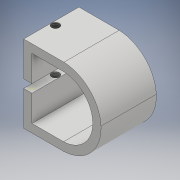
# Autodesk Inventor part: Goupille
Saved by Autodesk Inventor 2018.1 (Build 221171000, 171)
## iProperties
Created: 2019-11-08
Part Number: Goupille
Material: Générique
Document SubType Name: Modeling
Designer: tgremling1
Density: 1 g/cm^3
Appearance: Par défaut
Author: tgremling1
Autodesk Inventor part; units mm, degrees
ref_plane "YZ Plane" through (0, 0, 0) normal (1, 0, 0) x (0, 1, 0)
sketch "Esquisse1" plane through (0, 0, 0) normal (0, 1, 0) x (-1, 0, 0)
  line L0 (11, -11) -> (11, 11)
  arc A0 (-0.5, 11) -> (-11, -0.5) centre (-0.0119, 0.0108) ccw
  arc A1 (-11, 0.5) -> (0, -11) centre (-0.0114, 0) ccw
  line L1 (11, 11) -> (-0.5, 11)
  line L2 (11, -11) -> (-0.5, -11)
  arc A2 (-0.5626, 14) -> (-13.9968, -0.6393) centre (-0.0119, 0.0108) ccw
  line L3 (-0.5626, 14) -> (14, 14)
  line L4 (14, 14) -> (14, -14)
  line L5 (14, -14) -> (-0.5, -14)
  arc A3 (-13.9968, 0.661) -> (-0.5, -14) centre (0.0221, 0.0236) ccw
  point P0 (0, 0)
  point P1 (-11, 0)
  constraints: 12 end point, 9 point on circle, 4 centre point, 2 horizontal, 3 other
extrude "Extrusion1" add sketch "Esquisse1" along normal blind 20 contours L2 A1 A0 L1 L0 | L3 L4 L5 A3 A2
sketch "Esquisse2" plane through (0, 0, 0) normal (0, -1, 0) x (1, 0, 0)
  line L0 (13.9968, 0.661) -> (13.9968, 0.661)
  arc A0 (10.9999, 0.5232) -> (0.5, 11) centre (0.0119, 0.0108) ccw
  arc A1 (0.4408, -11) -> (10.9999, 0.5232) centre (-0.0221, 0.0236) ccw
  line L1 (0.4408, -11) -> (-11, -11)
  line L2 (-11, -11) -> (-11, 11)
  line L3 (-11, 11) -> (0.5, 11)
  point P0 (0, 0)
  constraints: 8 end point, 4 point on circle, 2 centre point
extrude "Extrusion2" cut sketch "Esquisse2" against normal blind 20
sketch "Esquisse3" plane through (-11, 0, 11) normal (1, 0, 0) x (0, 0, -1)
  point P0 (11, 0)
sketch "Esquisse4" plane through (0, 20, 0) normal (0, 1, 0) x (1, 0, 0)
  line L0 (-14, 1.5) -> (-11, 1.5)
  line L1 (-11, 1.5) -> (-11, -1.5)
  line L2 (-11, -1.5) -> (-14, -1.5)
  line L3 (-14, -1.5) -> (-14, 1.5)
  constraints: 8 end point, 2 parallel, 1 horizontal, 1 perpendicular
ref_plane "Plan de construction2" through (-14, 20, -1.5) normal (0, 0, 1) x (1, 0, 0)
ref_plane "Plan de construction3" through (-11, 20, 1.5) normal (0, 0, -1) x (-1, 0, 0)
extrude "Extrusion6" cut sketch "Esquisse4" against normal through all
sketch "Esquisse7" plane through (-11, 20, 1.5) normal (0, 0, -1) x (-1, 0, 0)
  line L0 (3, 0) -> (3, -20) projected
  line L1 (3, 0) -> (3, -10)
  line L2 (3, -10) -> (1.5, -10)
  circle A0 centre (1.5, -10) radius 1.375
  point P0 (-11, -20)
  dimension "d46" = 10
  dimension "d47" = 1.5
  dimension "d48" = 2.75
  constraints: 4 end point, 1 centre point, 1 coincident, 1 midpoint, 1 perpendicular
  measures "d46" distance of L0.start L1.end
  measures "d47" distance of L1.end L2.end
  measures "d48" diameter of A0
extrude "Extrusion7" cut sketch "Esquisse7" against normal through all
sketch "Esquisse8" plane through (-14, 20, -1.5) normal (0, 0, 1) x (1, 0, 0)
  line L0 (3, 0) -> (3, -10)
  line L1 (3, -10) -> (1.5, -10)
  circle A0 centre (1.5, -10) radius 1.375
  point P0 (-11, -20)
  dimension "d51" = 10
  dimension "d52" = 1.5
  dimension "d53" = 2.75
  constraints: 4 end point, 1 centre point, 1 coincident, 1 perpendicular
  measures "d51" distance of L0.start L0.end
  measures "d52" distance of L0.end L1.end
  measures "d53" diameter of A0
extrude "Extrusion9" cut sketch "Esquisse8" against normal blind 3
thread "Filetage1" size "M3x0.5" class "6H" standard "ANSI Metric M Profile" length 14.5
thread "Filetage2" size "M3x0.5" class "6H" standard "ANSI Metric M Profile" full length
thread "Filetage3" size "M3x0.5" class "6H" standard "ANSI Metric M Profile" length 3
